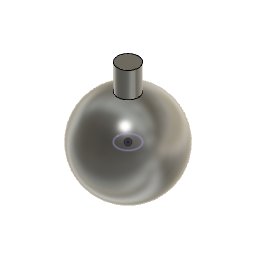
Foot_13mm v1 (Autodesk Fusion 360 design; units mm, degrees)
Autodesk Fusion 360 part; units mm, degrees
sketch "Sketch1" plane through (0, 0, 0) normal (0, 0, 1) x (1, 0, 0)
  circle A0 centre (0, 0) radius 1.5
  dimension "d1" = 3
  constraint coincident A0.centre origin
  measures "d1" diameter of A0
extrude "Extrude1" add sketch "Sketch1" along normal blind 4
ref_plane "WorkPlane1" through (0, 0, 1) normal (0, 0, -1) x (-1, 0, 0)
ref_plane "WorkPlane2" through (0, 0, -6) normal (0, 0, -1) x (-1, 0, 0)
sketch "Sketch2" plane through (0, 0, -6) normal (0, 0, -1) x (-1, 0, 0)
  circle A0 centre (0, 0) radius 1.5
  constraint coincident A0.centre origin
sphere "SpherePrimitive1" add diameter 13 placed x (-1, 0, 0) y (0, 1, 0) z (0, 0, -1) at (0, 0, -6)
